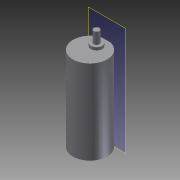
# Autodesk Inventor part: Hjul Motor
Saved by Autodesk Inventor 2012 SP1 (Build 160190100, 190)
## iProperties
Created: 2014-02-18
Part Number: Hjul Motor
Material: Default
Document SubType Name: Modeling
Designer: Pinkponk
Density: 1 g/cm^3
Author: Pinkponk
Autodesk Inventor part; units mm, degrees
ref_plane "YZ Plane" through (0, 0, 0) normal (1, 0, 0) x (0, 1, 0)
ref_plane "XY Plane" through (0, 0, 0) normal (0, 0, 1) x (1, 0, 0)
sketch "Sketch1" plane through (0, 0, 0) normal (0, 0, 1) x (1, 0, 0)
  circle A0 centre (0, 0) radius 15
  dimension "d0" = 30
  constraints: 1 centre point, 1 coincident
  measures "d0" diameter of A0
extrude "Extrusion1" add sketch "Sketch1" along normal blind 74
sketch "Sketch2" plane through (0, 0, 74) normal (0, 0, 1) x (1, 0, 0)
  circle A0 centre (0, 0) radius 15 projected
  circle A1 centre (0, 5.73) radius 5
  dimension "d3" = 10
  dimension "d4" = 15.73
  constraints: 1 centre point, 1 vertical alignment
  measures "d3" diameter of A1
extrude "Extrusion2" add sketch "Sketch2" along normal blind 2.5 contours A1
sketch "Sketch3" plane through (0, 5.73, 76.5) normal (0, 0, 1) x (1, 0, 0)
  circle A0 centre (0, 0) radius 5 projected
  circle A1 centre (0, 0) radius 2.5
  point P0 (0, -5.73)
  dimension "d7" = 5
  constraints: 1 centre point, 1 coincident
  measures "d7" diameter of A1
extrude "Extrusion3" add sketch "Sketch3" along normal blind 10 contours A1
sketch "Sketch4" plane through (0, 0, 0) normal (0, 1, 0) x (-1, 0, 0)
  point P0 (0, 0)
ref_plane "Work Plane1" through (0, 15, 0) normal (0, 1, 0) x (-1, 0, 0)
sketch "Sketch5" plane through (0, 15, 0) normal (0, 1, 0) x (-1, 0, 0)
  line L0 (-5, 74) -> (5, 74)
  line L1 (5, 74) -> (5, 72)
  line L2 (5, 72) -> (-5, 72)
  line L3 (-5, 72) -> (-5, 74)
  line L4 (-15, 74) -> (15, 74) projected
  point P0 (0, 0)
  point P1 (0, 74)
  dimension "d11" = 10
  dimension "d12" = 2
  constraints: 8 end point, 2 midpoint, 2 parallel, 1 horizontal, 1 perpendicular, 1 vertical alignment
  measures "d11" distance of L1.end L2.end
  measures "d12" distance of L0.end L1.end
extrude "Extrusion4" cut sketch "Sketch5" against normal blind 0.5
body "Solid1"
